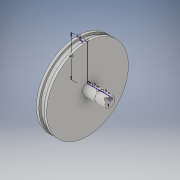
# Autodesk Inventor part: SpoolWinderDriver2
Saved by Autodesk Inventor 2019 (Build 230136000, 136)
## iProperties
Created: 2019-01-14
Part Number: SpoolWinderDriver2
Material: Generic
Document SubType Name: Modeling
Designer: Kepler
Density: 1 g/cm^3
Appearance: Default
Author: Kepler
Autodesk Inventor part; units mm, degrees
ref_plane "YZ Plane" through (0, 0, 0) normal (1, 0, 0) x (0, 1, 0)
ref_plane "XZ Plane" through (0, 0, 0) normal (0, 1, 0) x (-1, 0, 0)
ref_plane "XY Plane" through (0, 0, 0) normal (0, 0, 1) x (1, 0, 0)
sketch "Sketch1" plane through (0, 0, 0) normal (0, 0, 1) x (1, 0, 0)
  line L0 (0, 0) -> (0, 40)
  line L1 (0, 40) -> (2.5, 40)
  line L2 (2.5, 40) -> (2.5, 38)
  line L3 (2.5, 38) -> (7.5, 38)
  line L4 (7.5, 38) -> (7.5, 40)
  line L5 (7.5, 40) -> (10, 40)
  line L6 (10, 40) -> (10, 4.8)
  line L7 (10, 4.8) -> (22, 4.8)
  line L8 (22, 4.8) -> (22, 4.9)
  line L9 (22, 4.9) -> (32, 4.9)
  line L10 (32, 4.9) -> (32, 0)
  line L11 (32, 0) -> (0, 0)
  dimension "d0" = 40
  dimension "d1" = 2.5
  dimension "d2" = 2
  dimension "d3" = 5
  dimension "d4" = 2.5
  dimension "d6" = 12
  dimension "d7" = 0.1
  dimension "d8" = 10
  dimension "d11" = 9.8
  constraints: 24 end point, 7 perpendicular, 2 horizontal, 2 point on line, 2 vertical
  measures "d0" distance of L0.start L0.end
  measures "d1" distance of L0.end L1.end
  measures "d2" distance of L1.end L2.end
  measures "d3" distance of L2.end L3.end
  measures "d4" distance of L4.end L5.end
  measures "d6" distance of L6.end L7.end
  measures "d7" distance of L7.end L8.end
  measures "d8" distance of L8.end L9.end
  measures "d11" diameter of L9 L11
revolve "Revolution1" add sketch "Sketch1" angle 360 about axis through (32, 0, 0) along (-1, 0, 0)
body "Solid1"
